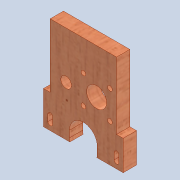
# Autodesk Inventor part: 0005-10-005
Saved by Autodesk Inventor 2020 (Build 240168000, 168)
## iProperties
Created: 2020-12-18
Part Number: 0005-10-005
Material: Generic
Document SubType Name: Modeling
Designer: Iulian Bors
Density: 1 g/cm^3
Appearance: White Oak - Natural Medium Gloss
Author: Iulian Bors
Subject: 005
Autodesk Inventor part; units mm, degrees
ref_plane "YZ Plane" through (0, 0, 0) normal (1, 0, 0) x (0, 1, 0)
ref_plane "XZ Plane" through (0, 0, 0) normal (0, 1, 0) x (-1, 0, 0)
ref_plane "XY Plane" through (0, 0, 0) normal (0, 0, 1) x (1, 0, 0)
sketch "Sketch1" plane through (0, 0, 0) normal (0, 0, 1) x (1, 0, 0)
  line L0 (-30, 32.5) -> (30, 32.5)
  line L1 (30, 32.5) -> (30, -32.5)
  line L2 (30, -32.5) -> (-30, -32.5)
  line L3 (-30, -32.5) -> (-30, 32.5)
  point P0 (0, 0)
  point P1 (0, 32.5)
  point P2 (-30, 0)
  dimension "d0" = 60
  dimension "d1" = 65
  constraints: 8 end point, 2 midpoint, 2 parallel, 1 horizontal, 1 horizontal alignment, 1 perpendicular, 1 vertical alignment
  measures "d0" distance of L0.start L0.end
  measures "d1" distance of L2.end L0.start
extrude "Extrusion1" add sketch "Sketch1" along normal blind 10
sketch "Sketch4" plane through (0, 0, 10) normal (0, 0, 1) x (1, 0, 0)
  circle A0 centre (-25, -15) radius 1.75
  circle A1 centre (25, -15) radius 1.75
  circle A2 centre (25, -25) radius 1.75
  arc A3 (-10.5, -30) -> (10.5, -30) centre (0, -30) ccw
  line L0 (10.5, -30) -> (10.5, -25)
  arc A4 (10.5, -25) -> (-10.5, -25) centre (0, -25) ccw
  line L1 (-10.5, -25) -> (-10.5, -30)
  line L2 (30, -10) -> (30, -50)
  line L3 (30, -50) -> (-30, -50)
  line L4 (-30, -50) -> (-30, -10)
  line L5 (-30, -10) -> (30, -10)
  line L6 (25, -27.5) -> (25, -22.5) construction
  line L7 (26.75, -27.5) -> (26.75, -22.5)
  line L8 (23.25, -22.5) -> (23.25, -27.5)
  arc A5 (23.25, -27.5) -> (26.75, -27.5) centre (25, -27.5) ccw
  arc A6 (26.75, -22.5) -> (23.25, -22.5) centre (25, -22.5) ccw
  line L9 (-25, -27.5) -> (-25, -22.5) construction
  line L10 (-23.25, -27.5) -> (-23.25, -22.5)
  line L11 (-26.75, -22.5) -> (-26.75, -27.5)
  arc A7 (-26.75, -27.5) -> (-23.25, -27.5) centre (-25, -27.5) ccw
  arc A8 (-23.25, -22.5) -> (-26.75, -22.5) centre (-25, -22.5) ccw
  line L12 (-30, -32.5) -> (30, -32.5) projected
  point P0 (0, 0)
  point P1 (-25, -25)
  point P2 (26.75, -25)
  point P3 (23.25, -25)
  dimension "d22" = 5
  dimension "d23" = 3.5
  dimension "d24" = 5
  dimension "d25" = 10.5
  dimension "d26" = 7.5
  dimension "d27" = 30
  constraints: 28 end point, 12 point on circle, 9 centre point, 8 tangent, 4 parallel, 3 vertical, 2 horizontal, 2 midpoint, 1 coincident, 1 equal radius, 1 horizontal alignment, 1 vertical alignment, 10 other
  measures "d22" distance of L6.start L6.end
  measures "d23" diameter of A6
  measures "d24" distance of A4.centre A3.centre
  measures "d25" radius of A4
  measures "d26" distance from line of A4.centre L12
  measures "d27" distance from line of L2 A3.centre
extrude "Extrusion4" cut sketch "Sketch4" against normal blind 10 contours A2 | L7 A5 L8 A2 | A2 L8 A6 L7 | L1 A4 L0 A3 L12 | L12 A3 | A7 L11 A8 L10
sketch "Sketch5" plane through (0, 0, 10) normal (0, 0, 1) x (1, 0, 0)
  circle A0 centre (10, 6.8914) radius 7.5
  line L0 (30, 32.5) -> (-30, 32.5) projected
  line L1 (30, -32.5) -> (30, 32.5) projected
  point P0 (0, 0)
  dimension "d13" = 15
  dimension "d28" = 25.6086
  dimension "d29" = 20
  constraints: 1 centre point
  measures "d13" diameter of A0
  measures "d28" distance from line of A0.centre L0
  measures "d29" distance from line of L1 A0.centre
extrude "Extrusion5" cut sketch "Sketch5" against normal through all
sketch "Sketch6" plane through (0, 0, 10) normal (0, 0, 1) x (1, 0, 0)
  circle A0 centre (20, 17.6414) radius 1.75
  circle A1 centre (0, 17.6414) radius 1.75
  circle A2 centre (0, -3.8586) radius 1.75
  circle A3 centre (20, -3.8586) radius 1.75
  line L0 (0, 17.6414) -> (20, 17.6414) construction
  line L1 (20, 17.6414) -> (20, -3.8586) construction
  line L2 (20, -3.8586) -> (0, -3.8586) construction
  line L3 (0, -3.8586) -> (0, 17.6414) construction
  line L4 (30, -32.5) -> (30, 32.5) construction
  line L5 (30, 32.5) -> (-30, 32.5) construction
  circle A4 centre (10, 6.8914) radius 7.5 projected
  point P0 (0, 0)
  point P1 (10, -3.8586)
  point P2 (20, 6.8914)
  dimension "d31" = 21.5
  dimension "d33" = 3.5
  dimension "d42" = 20
  constraints: 8 end point, 4 centre point, 3 equal radius, 2 coincident, 2 midpoint, 2 parallel, 1 horizontal, 1 horizontal alignment, 1 perpendicular, 1 vertical alignment
  measures "d31" distance of L2.end L0.start
  measures "d33" diameter of A1
  measures "d42" distance of L1.end L2.end
extrude "Extrusion6" cut sketch "Sketch6" against normal through all contours A0 | A1 | A2 | A3
sketch "Sketch7" plane through (0, 0, 10) normal (0, 0, 1) x (1, 0, 0)
  line L0 (-30, 32.5) -> (-30, -32.5) projected
  line L1 (-30, -7.5) -> (-25, -7.5)
  line L2 (-25, -7.5) -> (-25, 32.5)
  line L3 (-25, 32.5) -> (-30, 32.5)
  line L4 (-30, 32.5) -> (-30, -7.5)
  line L5 (30, 32.5) -> (-30, 32.5) projected
  line L6 (30, -10) -> (-30, -10) projected
  line L7 (25, -10) -> (30, -10)
  line L8 (30, -10) -> (30, 32.5)
  line L9 (30, 32.5) -> (25, 32.5)
  line L10 (25, 32.5) -> (25, -10)
  line L11 (30, -32.5) -> (30, 32.5) projected
  point P0 (0, 0)
  point P1 (25, -10)
  dimension "d18" = 5
  dimension "d19" = 5
  dimension "d43" = 40
  constraints: 16 end point, 4 collinear, 4 parallel, 2 horizontal, 2 perpendicular, 1 point on line
  measures "d18" distance between parallel lines of L2 L0
  measures "d19" distance between parallel lines of L8 L10
  measures "d43" distance of L1.end L2.end
extrude "Extrusion7" cut sketch "Sketch7" against normal through all contours L3 L2 L1 L0 | L5 L8 L6 L10
sketch "Sketch8" plane through (0, 0, 10) normal (0, 0, 1) x (1, 0, 0)
  circle A0 centre (-13, 5.0309) radius 4
  line L0 (-30, -7.5) -> (-30, -32.5) projected
  line L1 (25, 32.5) -> (-25, 32.5) projected
  point P0 (0, 0)
  dimension "d35" = 8
  dimension "d36" = 17
  dimension "d37" = 27.4691
  constraints: 1 centre point
  measures "d35" diameter of A0
  measures "d36" distance from line of A0.centre L0
  measures "d37" distance from line of A0.centre L1
extrude "Extrusion8" cut sketch "Sketch8" against normal blind 10
move faces "Move1" translate (0, 8, 0) faces at (8.3333, 32.5, 3.3333)
equation "\"d19\" = d18"
body "Solid1"
